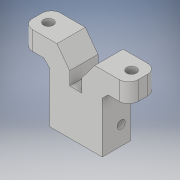
# Autodesk Inventor part: holder-GT2-x-carriage-left
Saved by Autodesk Inventor 2018 (Build 220112000, 112)
## iProperties
Created: 2017-10-15
Part Number: holder-GT2-x-carriage-left
Material: Generic
Document SubType Name: Modeling
Designer: Jurjen
Density: 1 g/cm^3
Appearance: Default
Author: Jurjen
Autodesk Inventor part; units mm, degrees
ref_plane "YZ Plane" through (0, 0, 0) normal (1, 0, 0) x (0, 1, 0)
ref_plane "XZ Plane" through (0, 0, 0) normal (0, 1, 0) x (-1, 0, 0)
ref_plane "XY Plane" through (0, 0, 0) normal (0, 0, 1) x (1, 0, 0)
sketch "Sketch1" plane through (0, 0, 0) normal (0, 0, 1) x (1, 0, 0)
  line L0 (-28, 25) -> (28, 25)
  line L1 (28, 25) -> (28, 15)
  line L2 (28, 15) -> (14, 15)
  line L3 (14, 15) -> (14, -15)
  line L4 (14, -15) -> (10, -15)
  line L5 (10, -15) -> (10, 15)
  line L6 (10, 15) -> (-10, 15)
  line L7 (-10, 15) -> (-10, -15)
  line L8 (-10, -15) -> (-14, -15)
  line L9 (-14, -15) -> (-14, 15)
  line L10 (-14, 15) -> (-28, 15)
  line L11 (-28, 15) -> (-28, 25)
  point P0 (0, 0)
  point P1 (0, 25)
  point P2 (0, 15)
  point P3 (10, 0)
  dimension "d0" = 20
  dimension "d1" = 30
  dimension "d2" = 4
  dimension "d3" = 4
  dimension "d4" = 14
  dimension "d5" = 10
  constraints: 24 end point, 8 perpendicular, 6 point on line, 3 midpoint, 2 vertical alignment, 1 horizontal, 1 horizontal alignment
  measures "d0" distance between parallel lines of L5 L7
  measures "d1" distance between parallel lines of L2 L4
  measures "d2" distance between parallel lines of L3 L5
  measures "d3" distance between parallel lines of L7 L9
  measures "d4" distance between parallel lines of L11 L9
  measures "d5" distance between parallel lines of L0 L2
extrude "Extrusion1" add sketch "Sketch1" along normal mid plane 15
sketch "Sketch2" plane through (-28, 25, 7.5) normal (0, 1, 0) x (1, 0, 0)
  circle A0 centre (6, 7.5) radius 2.6
  circle A1 centre (50, 7.5) radius 2.6
  line L0 (0, 15) -> (0, 0) projected
  line L1 (56, 0) -> (56, 15) projected
  point P0 (28, 7.5)
  dimension "d8" = 5.2
  dimension "d9" = 6
  dimension "d10" = 6
  constraints: 2 centre point, 2 horizontal alignment, 1 equal radius
  measures "d8" diameter of A0
  measures "d9" distance from line of L0 A0.centre
  measures "d10" distance from line of A1.centre L1
extrude "Extrusion2" cut sketch "Sketch2" against normal up to next
sketch "Sketch3" plane through (-28, 15, 7.5) normal (0, -1, 0) x (1, 0, 0)
  circle A0 centre (6, -7.5) radius 2.6 projected
  circle A1 centre (50, -7.5) radius 2.6 projected
  line L0 (1.9, -10.2201) -> (1.9, -4.7799)
  line L1 (1.9, -4.7799) -> (6, -3.05)
  line L2 (6, -3.05) -> (10.1, -4.7799)
  line L3 (10.1, -4.7799) -> (10.1, -10.2201)
  line L4 (14, 0) -> (14, -15) projected
  line L5 (10.1, -10.2201) -> (6, -11.95)
  line L6 (6, -11.95) -> (1.9, -10.2201)
  point P0 (28, -7.5)
  point P1 (1.9, -7.5)
  dimension "d13" = 8.2
  dimension "d22" = 8.9
  dimension "d23" = 8.2
  constraints: 12 end point, 3 horizontal alignment, 3 parallel, 3 vertical alignment, 1 midpoint, 1 vertical
  measures "d13" distance between parallel lines of L3 L0
  measures "d22" distance of L1.end L5.end
  measures "d23" distance between parallel lines of L6 L2
extrude "Extrusion3" cut sketch "Sketch3" against normal blind 5 contours L0 L1 L2 L3 L5 L6
mirror "Mirror1" about plane through (0, 0, 0) normal (1, 0, 0) of "Extrusion3"
sketch "Sketch4" plane through (14, -15, 7.5) normal (1, 0, 0) x (0, 0, -1)
  circle A0 centre (10, 10) radius 2.1
  line L0 (0, 0) -> (15, 0) projected
  point P0 (7.5, 15)
  point P1 (7.5, 0)
  point P2 (7.5, 0)
  dimension "d24" = 4.2
  dimension "d25" = 10
  constraints: 2 midpoint, 2 vertical alignment, 1 centre point
  measures "d24" diameter of A0
  measures "d25" distance from line of A0.centre L0
extrude "Extrusion4" cut sketch "Sketch4" against normal up to surface (28 mm away)
fillet "Fillet1" radius 5 4 edges at (-28, 20, 7.5) (-28, 20, -7.5) (28, 20, 7.5) (28, 20, -7.5)
chamfer "Chamfer1" distance 3 angle 45 2 edges at (-14, 15, 0) (14, 15, 0)
sketch "Sketch8" plane through (0, 0, 7.5) normal (0, 0, 1) x (1, 0, 0)
  line L0 (-10, 15) -> (10, 15)
  line L1 (10, 15) -> (10, -15)
  line L2 (10, -15) -> (-10, -15)
  line L3 (-10, -15) -> (-10, 15)
  point P0 (0, 0)
  constraints: 8 end point, 2 parallel, 1 horizontal, 1 perpendicular
extrude "Extrusion7" add sketch "Sketch8" against normal blind 3
sketch "Sketch9" plane through (0, 0, -7.5) normal (0, 0, -1) x (-1, 0, 0)
  line L0 (-10, 5) -> (10, 5)
  line L1 (10, -15) -> (14, -15) projected
  line L2 (-10, 5) -> (-10, 15)
  line L3 (-10, 15) -> (10, 15)
  line L4 (10, 15) -> (10, 5)
  point P0 (0, 0)
  dimension "d44" = 20
  constraints: 8 end point, 2 perpendicular, 2 vertical alignment, 1 horizontal, 1 vertical
  measures "d44" distance between parallel lines of L1 L0
extrude "Extrusion8" add sketch "Sketch9" against normal up to surface (12 mm away)
sketch "Sketch6" plane through (0, 0, 7.5) normal (0, 0, 1) x (1, 0, 0)
  line L0 (-3.25, 16) -> (3.25, 16)
  line L1 (3.25, 16) -> (10, 25)
  line L2 (28, 25) -> (-28, 25) projected
  line L3 (-3.25, 16) -> (-10, 25)
  line L4 (-10, 25) -> (10, 25)
  line L5 (-14, -15) -> (-10, -15) projected
  line L6 (-10, 5) -> (10, 5) projected
  line L7 (-3.25, 16) -> (-3.25, 9)
  line L8 (-3.25, 9) -> (3.25, 9)
  line L9 (3.25, 9) -> (3.25, 16)
  point P0 (0, 0)
  point P1 (0, 16)
  point P2 (0, 25)
  point P3 (-10, 15)
  point P4 (0, 25)
  point P5 (0, 25)
  dimension "d29" = 6.5
  dimension "d30" = 20
  dimension "d47" = 9
  dimension "d48" = 4
  constraints: 14 end point, 4 midpoint, 3 perpendicular, 2 point on line, 1 coincident, 1 collinear, 1 horizontal, 1 vertical alignment
  measures "d29" distance of L0.start L0.end
  measures "d30" distance of L1.end L3.end
  measures "d47" distance between parallel lines of L2 L0
  measures "d48" distance between parallel lines of L6 L8
extrude "Extrusion5" cut sketch "Sketch6" against normal up to surface (15 mm away)
sketch "Sketch11" plane through (-3.25, 9, 7.5) normal (0, 1, 0) x (1, 0, 0)
  line L0 (13.25, 7.9) -> (13.25, 12.1) projected
  line L1 (17.25, 12.1) -> (17.25, 7.9) projected
  circle A0 centre (3.25, 10) radius 2.1
  point P0 (3.25, 7.5)
  point P1 (17.25, 10)
  dimension "d49" = 4.2
  constraints: 1 centre point, 1 horizontal alignment, 1 midpoint, 1 vertical alignment
  measures "d49" diameter of A0
extrude "Extrusion9" cut sketch "Sketch11" against normal up to next
equation "\"d3\" = d2"
body "Solid1"
